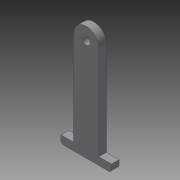
# Autodesk Inventor part: arm3
Saved by Autodesk Inventor 2015 (Build 190159000, 159)
## iProperties
Created: 2015-06-16
Part Number: arm3
Material: Generic
Document SubType Name: Modeling
Designer: Robert Allen Fett
Density: 1 g/cm^3
Appearance: Default
Author: Robert Allen Fett
Autodesk Inventor part; units mm, degrees
ref_plane "YZ Plane" through (0, 0, 0) normal (1, 0, 0) x (0, 1, 0)
ref_plane "XZ Plane" through (0, 0, 0) normal (0, 1, 0) x (-1, 0, 0)
ref_plane "XY Plane" through (0, 0, 0) normal (0, 0, 1) x (1, 0, 0)
sketch "Sketch1" plane through (0, 0, 0) normal (0, 0, 1) x (1, 0, 0)
  line L0 (5, -6) -> (-5, -6)
  circle A0 centre (0, 31.25) radius 1.5
  arc A1 (5, 31.25) -> (-5, 31.25) centre (0, 31.25) ccw
  line L1 (-5, -6) -> (-5, 31.25)
  line L2 (5, -6) -> (5, 31.25)
  point P0 (0, 0)
  point P1 (0, 0)
  point P2 (0, -6)
  point P3 (0, -6)
  dimension "d2" = 3
  dimension "d13" = 10
  dimension "d15" = 37.25
  dimension "d16" = 6
  constraints: 6 end point, 3 vertical alignment, 2 centre point, 2 midpoint, 2 point on circle, 2 tangent, 1 coincident, 1 horizontal, 1 parallel
  measures "d2" diameter of A0
  measures "d13" distance between parallel lines of L2 L1
  measures "d15" distance from line of L0 A0.centre
  measures "d16" distance from line of L0 point (0, 0)
extrude "Extrusion1" add sketch "Sketch1" along normal blind 3
sketch "Sketch2" plane through (0, 0, 3) normal (0, 0, 1) x (1, 0, 0)
  line L0 (10, -6) -> (10, -9)
  line L1 (10, -9) -> (-10, -9)
  line L2 (-5, -6) -> (5, -6) projected
  line L3 (5, -6) -> (5, 31.25) projected
  line L4 (10, -6) -> (-10, -6)
  line L5 (-10, -6) -> (-10, -9)
  line L6 (-5, 31.25) -> (-5, -6) projected
  point P0 (0, 0)
  dimension "d5" = 3
  dimension "d17" = 5
  dimension "d18" = 5
  constraints: 8 end point, 1 collinear, 1 horizontal, 1 parallel, 1 perpendicular
  measures "d5" distance of L0.start L0.end
  measures "d17" distance between parallel lines of L0 L3
  measures "d18" distance between parallel lines of L5 L6
extrude "Extrusion2" add sketch "Sketch2" against normal blind 3
fillet "Fillet1" radius 1 2 edges at (-10, -9, 1.5) (10, -9, 1.5)
body "Solid1"
